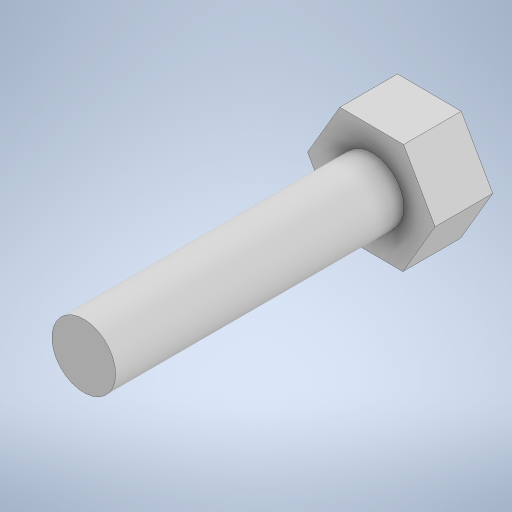
# Autodesk Inventor part: nut
Saved by Autodesk Inventor 2023 (Build 270158000, 158)
## iProperties
Created: 2022-06-19
Part Number: nut
Material: Generic
Document SubType Name: Modeling
Designer: ADITYA CHINAGUDI
Density: 1 g/cm^3
Appearance: Default
Author: ADITYA CHINAGUDI
Autodesk Inventor part; units mm, degrees
ref_plane "YZ Plane" through (0, 0, 0) normal (1, 0, 0) x (0, 1, 0)
ref_plane "XZ Plane" through (0, 0, 0) normal (0, 1, 0) x (-1, 0, 0)
ref_plane "XY Plane" through (0, 0, 0) normal (0, 0, 1) x (1, 0, 0)
sketch "Sketch1" plane through (0, 0, 0) normal (0, 0, 1) x (1, 0, 0)
  line L0 (-1.3324, 3.0361) -> (-3.5431, 3.0514)
  line L1 (-3.5431, 3.0514) -> (-4.6352, 4.9735)
  line L2 (-4.6352, 4.9735) -> (-3.5166, 6.8804)
  line L3 (-3.5166, 6.8804) -> (-1.306, 6.8651)
  line L4 (-1.306, 6.8651) -> (-0.2138, 4.943)
  line L5 (-0.2138, 4.943) -> (-1.3324, 3.0361)
  point P0 (0, 0)
  point P1 (-2.4245, 4.9582)
  constraints: 12 end point, 13 other
extrude "Extrusion1" add sketch "Sketch1" along normal blind 2
sketch "Sketch2" plane through (0, 0, 2) normal (0, 0, 1) x (1, 0, 0)
  circle A0 centre (-2.3976, 4.9735) radius 1.1054
  point P0 (0, 0)
  constraints: 1 centre point
extrude "Extrusion2" add sketch "Sketch2" along normal blind 10
body "Solid1"
